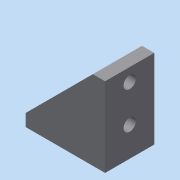
# Autodesk Inventor part: corners
Saved by Autodesk Inventor 2015 (Build 190159000, 159)
## iProperties
Created: 2016-06-24
Part Number: corners
Material: Generic
Document SubType Name: Modeling
Designer: Dustin
Density: 1 g/cm^3
Appearance: Default
Author: Dustin
Autodesk Inventor part; units mm, degrees
ref_plane "YZ Plane" through (0, 0, 0) normal (1, 0, 0) x (0, 1, 0)
ref_plane "XZ Plane" through (0, 0, 0) normal (0, 1, 0) x (-1, 0, 0)
ref_plane "XY Plane" through (0, 0, 0) normal (0, 0, 1) x (1, 0, 0)
sketch "Sketch1" plane through (0, 0, 0) normal (0, 0, 1) x (1, 0, 0)
  line L0 (0, 0) -> (50, 0)
  line L1 (50, 0) -> (50, 50)
  line L2 (50, 50) -> (0, 0)
  dimension "d0" = 50
  dimension "d1" = 50
  constraints: 6 end point, 1 horizontal, 1 perpendicular
  measures "d0" distance of L0.end L1.end
  measures "d1" distance of L0.start L0.end
extrude "Extrusion1" add sketch "Sketch1" along normal blind 20
sketch "Sketch2" plane through (0, 0, 20) normal (0, 0, 1) x (1, 0, 0)
  line L0 (50, 50) -> (0, 0) projected
  line L1 (5, 5) -> (45, 5)
  line L2 (45, 5) -> (45, 45)
  line L3 (50, 0) -> (50, 50) projected
  line L4 (0, 0) -> (50, 0) projected
  dimension "d4" = 5
  dimension "d5" = 5
  constraints: 4 end point, 2 point on line, 1 horizontal, 1 perpendicular
  measures "d4" distance between parallel lines of L3 L2
  measures "d5" distance between parallel lines of L4 L1
extrude "Extrusion2" cut sketch "Sketch2" against normal through all contours L2 L1 L0
extrude "Extrusion3" add sketch "Sketch2" against normal blind 5 contours L2 L1 L0
sketch "Sketch3" plane through (0, 0, 0) normal (0, 0, -1) x (-1, 0, 0)
  line L0 (-12.7, 0) -> (-50, 37.3)
  line L1 (-50, 0) -> (-50, 50) projected
  line L2 (-60.6675, 53.6604) -> (-50, 37.3)
  line L3 (-60.6675, 53.6604) -> (-37.4752, 61.571)
  line L4 (-37.4752, 61.571) -> (23.8314, -5.4888)
  line L5 (23.8314, -5.4888) -> (-5.9204, -12.6802)
  line L6 (-5.9204, -12.6802) -> (-12.7, 0)
  point P0 (0, 0)
  dimension "d12" = 12.7
  dimension "d13" = 12.7
  constraints: 12 end point, 1 point on line
  measures "d12" distance of L1.end L0.end
  measures "d13" distance of point (0, 0) L0.start
extrude "Extrusion5" cut sketch "Sketch3" against normal through all
sketch "Sketch5" plane through (45, 5, 0) normal (-1, 0, 0) x (0, 0, 1)
  line L0 (0, 0) -> (0, 27.3) projected
  line L1 (20, -5) -> (0, -5) projected
  point P0 (10, 22)
  point P1 (10, 7)
  dimension "d28" = 10
  dimension "d29" = 10
  dimension "d30" = 15
  dimension "d31" = 12
  measures "d28" distance from line of L0 point (10, 7)
  measures "d29" distance from line of L0 point (10, 22)
  measures "d30" distance of point (10, 7) point (10, 22)
  measures "d31" distance from line of L1 point (10, 7)
hole "Hole2" at (45, 27, 10) at (45, 12, 10) direction (1, 0, 0) diameter 5 depth 25.4 tip angle 118
sketch "Sketch6" plane through (45, 5, 15) normal (0, 1, 0) x (1, 0, 0)
  line L0 (-27.3, 15) -> (0, 15) projected
  line L1 (5, 15) -> (5, -5) projected
  point P0 (-45, 15)
  point P1 (-7, 5)
  point P2 (-22, 5)
  dimension "d39" = 15
  dimension "d40" = 10
  dimension "d41" = 10
  dimension "d42" = 12
  measures "d39" distance of point (-7, 5) point (-22, 5)
  measures "d40" distance from line of L0 point (-7, 5)
  measures "d41" distance from line of L0 point (-22, 5)
  measures "d42" distance from line of L1 point (-7, 5)
hole "Hole3" at (38, 5, 10) at (23, 5, 10) direction (0, -1, 0) diameter 5 depth 25.4 tip angle 118
sketch "Sketch7" plane through (0, 0, 0) normal (0, 0, -1) x (-1, 0, 0)
  line L0 (-17.7, 5) -> (-17.7, 0)
  line L1 (-12.7, 0) -> (-50, 0) projected
  line L2 (-17.7, 0) -> (-12.7, 0)
  line L3 (-12.7, 0) -> (-17.7, 5)
  line L4 (-12.7, 0) -> (-17.7, 5) projected
  line L5 (-45, 32.3) -> (-50, 32.3)
  line L6 (-50, 0) -> (-50, 37.3) projected
  line L7 (-50, 32.3) -> (-50, 37.3)
  line L8 (-50, 37.3) -> (-45, 32.3)
  line L9 (-45, 32.3) -> (-50, 37.3) projected
  point P0 (0, 0)
  constraints: 12 end point, 3 collinear, 2 horizontal, 2 point on line, 1 vertical
extrude "Extrusion6" cut sketch "Sketch7" against normal blind 25.4
body "Solid1"
